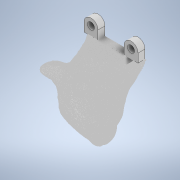
# Autodesk Inventor part: squirrel_head_small_dense
Saved by Autodesk Inventor 2020 (Build 240168000, 168)
## iProperties
Created: 2019-05-04
Part Number: squirrel_head_small_dense
Material: Generic
Document SubType Name: Modeling
Designer: mfans
Density: 1 g/cm^3
Appearance: Default
Author: mfans
Autodesk Inventor part; units mm, degrees
ref_plane "YZ Plane" through (0, 0, 0) normal (1, 0, 0) x (0, 1, 0)
ref_plane "XZ Plane" through (0, 0, 0) normal (0, 1, 0) x (-1, 0, 0)
ref_plane "XY Plane" through (0, 0, 0) normal (0, 0, 1) x (1, 0, 0)
sketch "Sketch1" plane through (-16.3672, -29.0933, 43.6298) normal (0, 0, -1) x (-1, 0, 0)
  line L0 (-25.3672, 15.6523) -> (-19.3672, 15.6523)
  line L1 (-19.3672, 15.6523) -> (-19.3672, 23.6523)
  line L2 (-19.3672, 23.6523) -> (-25.3672, 23.6523)
  line L3 (-25.3672, 23.6523) -> (-25.3672, 15.6523)
  line L4 (-2.3672, 23.6523) -> (3.6328, 23.6523)
  line L5 (3.6328, 23.6523) -> (3.6328, 15.6523)
  line L6 (3.6328, 15.6523) -> (-2.3672, 15.6523)
  line L7 (-2.3672, 15.6523) -> (-2.3672, 23.6523)
  point P0 (-16.3672, 29.0933)
  dimension "d0" = 6
  dimension "d1" = 8
  dimension "d2" = 0
  dimension "d4" = 17
  dimension "d5" = 3
  dimension "d20" = 13.441
  constraints: 16 end point, 4 parallel, 2 equal length, 2 horizontal, 2 perpendicular
  measures "d0" distance of L1.end L2.end
  measures "d1" distance of L2.end L0.start
  measures "d2" distance between parallel lines of L4 L2
  measures "d4" distance between parallel lines of L7 L1
  measures "d5" distance from line of point (-16.367, 29.093) L1
  measures "d20" distance from line of point (-16.367, 29.093) L0
extrude "Extrusion1" add sketch "Sketch1" against normal blind 4
fillet "Fillet1" radius 3 4 edges at (9, -5.441, 45.6298) (3, -5.441, 45.6298) (-14, -5.441, 45.6298) (-20, -5.441, 45.6298)
sketch "Sketch2" plane through (-16.3672, -29.0933, 47.6298) normal (0, 0, 1) x (1, 0, 0)
  arc A0 (25.3672, 20.6523) -> (19.3672, 20.6523) centre (22.3672, 20.6523) ccw projected
  line L0 (19.3672, 20.6523) -> (19.3672, 15.6523) projected
  line L1 (19.3672, 15.6523) -> (25.3672, 15.6523) projected
  line L2 (25.3672, 15.6523) -> (25.3672, 20.6523) projected
  arc A1 (2.3672, 20.6523) -> (-3.6328, 20.6523) centre (-0.6328, 20.6523) ccw projected
  line L3 (-3.6328, 20.6523) -> (-3.6328, 15.6523) projected
  line L4 (-3.6328, 15.6523) -> (2.3672, 15.6523) projected
  line L5 (2.3672, 15.6523) -> (2.3672, 20.6523) projected
  point P0 (16.3672, 29.0933)
  constraints: 2 coincident
hole "Hole1" at (6, -8.441, 47.6298) at (-17, -8.441, 47.6298) direction (0, 0, -1) diameter 4 end through all
thicken "Thicken1" operation add thickness 1 both sides no extend neighbours yes toward (0.2947552, 0.9555728, 0) faces at (6.8843, -5.5743, 44.9631) (6, -5.441, 44.9631) (3.8008, -6.4004, 44.9631)
thicken "Thicken2" operation add thickness 1 both sides no extend neighbours yes toward (0.0747301, 0.9972038, 0) faces at (-16.7757, -5.4494, 44.9631) (-17, -5.441, 44.9631) (-19.9916, -8.2167, 44.9631)
sketch "Sketch3" plane through (-9.7038, -13.4415, 54.1536) normal (0, 1, 0) x (-1, 0, 0)
  line L0 (11.2962, -6.5238) -> (3.2962, -6.5238) projected
  line L1 (-11.7038, -10.5238) -> (-19.7038, -10.5238) projected
  line L2 (4.3739, -6.5238) -> (-13.1102, -6.5238)
  line L3 (-13.1102, -6.5238) -> (-13.1102, -10.5238)
  line L4 (-13.1102, -10.5238) -> (4.3739, -10.5238)
  line L5 (4.3739, -10.5238) -> (4.3739, -6.5238)
  point P0 (-9.7038, -54.1536)
  constraints: 8 end point, 2 parallel, 2 point on line, 1 horizontal, 1 perpendicular
extrude "Extrusion2" add sketch "Sketch3" against normal blind 4
body "Solid1"
